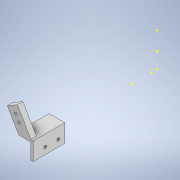
# Autodesk Inventor part: Bracket
Saved by Autodesk Inventor 2020.2 (Build 242310000, 310)
## iProperties
Created: 2020-10-07
Part Number: Bracket
Material: Generic
Document SubType Name: Modeling
Designer: Owner
Density: 1 g/cm^3
Appearance: Default
Author: Owner
Autodesk Inventor part; units mm, degrees
ref_plane "YZ Plane" through (0, 0, 0) normal (1, 0, 0) x (0, 1, 0)
ref_plane "XZ Plane" through (0, 0, 0) normal (0, 1, 0) x (-1, 0, 0)
ref_plane "XY Plane" through (0, 0, 0) normal (0, 0, 1) x (1, 0, 0)
sketch "Sketch1" plane through (0, 0, 0) normal (0, 0, 1) x (1, 0, 0)
  line L0 (0, 0) -> (19.05, 0)
  line L1 (19.05, 0) -> (19.05, 19.05)
  line L2 (19.05, 19.05) -> (0, 19.05)
  line L3 (0, 19.05) -> (0, 0)
  line L4 (19.05, 0) -> (22.225, 0)
  line L5 (22.225, 0) -> (22.225, 19.05)
  line L6 (22.225, 19.05) -> (19.05, 19.05)
  line L7 (19.05, 19.05) -> (19.05, 0)
  line L8 (0, 19.05) -> (22.225, 19.05)
  line L9 (22.225, 19.05) -> (22.225, 22.225)
  line L10 (22.225, 22.225) -> (0, 22.225)
  line L11 (0, 22.225) -> (0, 19.05)
  line L12 (0, 19.05) -> (-127, 19.05)
  line L13 (-127, 19.05) -> (-127, 22.225)
  line L14 (-127, 22.225) -> (0, 22.225)
  line L15 (0, 22.225) -> (0, 19.05)
  dimension "d0" = 19.05
  dimension "d1" = 19.05
  dimension "d2" = 3.175
  dimension "d3" = 3.175
  dimension "d4" = 127
  constraints: 32 end point, 8 parallel, 4 horizontal, 4 perpendicular, 2 point on line
  measures "d0" distance of L2.end L1.end
  measures "d1" distance of L1.end L0.end
  measures "d2" distance of L6.end L5.end
  measures "d3" distance of L9.end L8.end
  measures "d4" distance of L13.end L14.end
extrude "Extrusion1" add sketch "Sketch1" along normal blind 196.85 contours L1 L6 L5 L4 | L11 L10 L9 L6 L2 | L12 L13 L14 L11
sketch "Sketch2" plane through (-127, 22.225, 0) normal (0, 1, 0) x (1, 0, 0)
  line L0 (0, 0) -> (127, 0)
  line L1 (127, 0) -> (127, -34.925)
  line L2 (127, -34.925) -> (0, -34.925)
  line L3 (0, -34.925) -> (0, 0)
  dimension "d7" = 34.925
  constraints: 8 end point, 2 parallel, 1 horizontal, 1 perpendicular
  measures "d7" distance of L0.end L1.end
extrude "Extrusion2" cut sketch "Sketch2" against normal blind 25.4
sketch "Sketch3" plane through (-127, 22.225, 196.85) normal (0, 1, 0) x (1, 0, 0)
  line L0 (127, 161.925) -> (0, 161.925) projected
  line L1 (0, 161.925) -> (127, 161.925)
  line L2 (127, 161.925) -> (127, 158.75)
  line L3 (127, 158.75) -> (0, 158.75)
  line L4 (0, 158.75) -> (0, 161.925)
  point P0 (127, 196.85)
  dimension "d10" = 3.175
  constraints: 8 end point, 2 parallel, 1 horizontal, 1 perpendicular
  measures "d10" distance of L1.end L2.end
extrude "Extrusion3" add sketch "Sketch3" along normal blind 25.4
sketch "Sketch4" plane through (-127, 22.225, 196.85) normal (0, 1, 0) x (1, 0, 0)
  line L0 (149.225, 196.85) -> (127, 196.85) projected
  line L1 (149.225, 196.85) -> (149.225, 0) projected
  line L2 (127, 196.85) -> (149.225, 196.85)
  line L3 (149.225, 196.85) -> (149.225, 0)
  line L4 (149.225, 0) -> (127, 0)
  line L5 (127, 0) -> (127, 196.85)
  line L6 (149.225, 0) -> (0, 0) projected
  line L7 (138.1125, 0) -> (138.1125, 196.85)
  line L8 (127, 34.925) -> (149.225, 34.925)
  line L9 (127, 34.925) -> (149.225, 0)
  line L10 (127, 0) -> (149.225, 34.925)
  line L11 (127, 10.3909) -> (149.225, 24.5341)
  line L12 (127, 24.5341) -> (149.225, 10.3909)
  line L13 (127, 196.85) -> (127, 161.925) projected
  line L14 (127, 161.925) -> (149.225, 161.925)
  line L15 (127, 161.925) -> (149.225, 196.85)
  line L16 (149.225, 161.925) -> (127, 196.85)
  line L17 (127, 196.85) -> (127, 172.3159)
  line L18 (149.225, 186.4591) -> (127, 172.3159)
  line L19 (149.225, 172.3159) -> (127, 186.4591)
  line L20 (127, 186.4591) -> (149.225, 186.4591)
  line L21 (127, 10.3909) -> (149.225, 10.3909)
  line L22 (127, 172.3159) -> (149.225, 172.3159)
  line L23 (127, 24.5341) -> (149.225, 24.5341)
  circle A0 centre (138.1125, 10.3909) radius 1.905
  circle A1 centre (138.1125, 24.5341) radius 1.905
  circle A2 centre (138.1125, 172.3159) radius 1.905
  circle A3 centre (138.1125, 186.4591) radius 1.905
  dimension "d13" = 3.81
  dimension "d14" = 3.81
  dimension "d15" = 3.81
  dimension "d16" = 3.81
  constraints: 40 end point, 12 point on line, 11 perpendicular, 5 midpoint, 4 centre point, 3 parallel, 2 horizontal
  measures "d13" diameter of A0
  measures "d14" diameter of A1
  measures "d15" diameter of A2
  measures "d16" diameter of A3
extrude "Extrusion4" cut sketch "Sketch4" against normal blind 25.4 contours A3 L20 L7 | L7 L20 A3 | A3 L7 L20 | L7 A3 L20 | A2 L22 L7 | L7 L22 A2 | A2 L7 L22 | L7 A2 L22 | A1 L23 L7 | L7 L23 A1 | A1 L7 L23 | A0 L21 L7 | L7 L21 A0 | A1 L23 L7 | A0 L7 L21 | L7 A0 L21
sketch "Sketch5" plane through (22.225, 0, 0) normal (1, 0, 0) x (0, 0, -1)
  line L0 (0, 22.225) -> (-196.85, 22.225) projected
  line L1 (0, 0) -> (-196.85, 0) projected
  line L2 (-34.925, 22.225) -> (0, 22.225)
  line L3 (0, 22.225) -> (0, 0)
  line L4 (0, 0) -> (-34.925, 0)
  line L5 (-34.925, 0) -> (-34.925, 22.225)
  line L6 (-196.85, 22.225) -> (-161.925, 22.225)
  line L7 (-161.925, 22.225) -> (-161.925, 0)
  line L8 (-161.925, 0) -> (-196.85, 0)
  line L9 (-196.85, 0) -> (-196.85, 22.225)
  line L10 (-196.85, 19.05) -> (-196.85, 0) projected
  line L11 (-196.85, 11.1125) -> (0, 11.1125)
  line L12 (0, 19.05) -> (0, 0) projected
  line L13 (0, 22.225) -> (-34.925, 0)
  line L14 (-34.925, 22.225) -> (0, 0)
  line L15 (-196.85, 22.225) -> (-161.925, 0)
  line L16 (-161.925, 22.225) -> (-196.85, 0)
  line L17 (-186.4591, 22.225) -> (-172.3159, 0)
  line L18 (-174.2209, 22.225) -> (-170.4109, 22.225) projected
  line L19 (-172.3159, 22.225) -> (-186.4591, 0)
  line L20 (-24.4964, 22.225) -> (-10.3532, 0)
  line L21 (-10.3532, 22.225) -> (-24.4964, 0)
  line L22 (-24.4964, 22.225) -> (-24.4964, 0)
  line L23 (-10.3532, 22.225) -> (-10.3532, 0)
  line L24 (-186.4591, 22.225) -> (-186.4591, 0)
  line L25 (-172.3159, 22.225) -> (-172.3159, 0)
  circle A0 centre (-186.4591, 11.1125) radius 1.905
  circle A1 centre (-172.3159, 11.1125) radius 1.905
  circle A2 centre (-24.4964, 11.1125) radius 1.905
  dimension "d19" = 34.925
  dimension "d20" = 3.81
  dimension "d21" = 3.81
  dimension "d22" = 3.81
  constraints: 42 end point, 12 point on line, 11 parallel, 6 perpendicular, 4 midpoint, 3 centre point, 2 horizontal
  measures "d19" distance of L7.end L8.end
  measures "d20" diameter of A0
  measures "d21" diameter of A1
  measures "d22" diameter of A2
extrude "Extrusion5" cut sketch "Sketch5" against normal blind 25.4 contours A2 L11 L22 | L22 L11 A2 | L11 L22 A2 | A2 L22 L11 | A1 L25 L11 | L11 L25 A1 | L25 L11 A1 | L25 A1 L11 | A0 L24 L11 | L11 L24 A0 | L24 A0 L11 | L11 A0 L24
sketch "Sketch6" plane through (22.225, 0, 0) normal (1, 0, 0) x (0, 0, -1)
  line L0 (0, 22.225) -> (-196.85, 22.225) projected
  line L1 (0, 19.05) -> (0, 0) projected
  line L2 (-34.4902, 22.225) -> (0, 22.225)
  line L3 (0, 22.225) -> (0, 0)
  line L4 (0, 0) -> (-34.4902, 0)
  line L5 (-34.4902, 0) -> (-34.4902, 22.225)
  line L6 (-34.4902, 11.1125) -> (0, 11.1125)
  line L7 (0, 0) -> (0, 22.225) projected
  line L8 (0, 22.225) -> (-34.4902, 0)
  line L9 (-24.4058, 22.225) -> (-10.0843, 0)
  line L10 (0, 0) -> (-196.85, 0) projected
  line L11 (-10.0843, 0) -> (-10.0843, 22.225)
  circle A0 centre (-10.0843, 11.1125) radius 1.905
  dimension "d25" = 3.81
  constraints: 16 end point, 4 point on line, 3 midpoint, 3 perpendicular, 2 parallel, 1 centre point, 1 horizontal
  measures "d25" diameter of A0
extrude "Extrusion6" cut sketch "Sketch6" against normal blind 25.4 contours A0 L6 L11 | L11 L6 A0 | A0 L11 L6 | L6 L11 A0
sketch "Sketch7" plane through (0, 19.05, 34.925) normal (0, 0, -1) x (-1, 0, 0)
  point P0 (0, -19.05)
sketch "Sketch8" plane through (0, 19.05, 34.925) normal (0, 0, -1) x (-1, 0, 0)
  line L0 (0, 28.575) -> (127, 28.575) projected
  line L1 (0, 3.3903) -> (127, 3.3903)
  line L2 (127, 3.3903) -> (127, 28.575)
  line L3 (127, 28.575) -> (0, 28.575)
  line L4 (0, 28.575) -> (0, 3.3903)
  point P0 (0, -19.05)
  constraints: 8 end point, 2 parallel, 1 horizontal, 1 perpendicular
extrude "Extrusion7" cut sketch "Sketch8" against normal blind 25.4
sketch "Sketch9" plane through (-127, 22.225, 196.85) normal (0, 1, 0) x (1, 0, 0)
  point P0 (127, 196.85)
sketch "Sketch10" plane through (0, 19.05, 34.925) normal (0, 0, -1) x (-1, 0, 0)
  line L0 (0, 3.175) -> (0, 0) projected
  line L1 (0, 0) -> (127, 0)
  line L2 (127, 0) -> (127, 3.175)
  line L3 (127, 3.175) -> (0, 3.175)
  line L4 (0, 3.175) -> (0, 0)
  point P0 (0, -19.05)
  constraints: 8 end point, 2 parallel, 1 horizontal, 1 perpendicular
extrude "Extrusion8" cut sketch "Sketch10" against normal blind 184.15
sketch "Sketch11" plane through (0, 22.4403, 34.925) normal (0, 0, -1) x (-1, 0, 0)
  point P0 (0, -22.4403)
sketch "Sketch12" plane through (0, 22.4403, 34.925) normal (0, 0, -1) x (-1, 0, 0)
  line L0 (0, -3.3903) -> (0, -0.2153) projected
  line L1 (0, -3.3903) -> (693.4588, -3.3903)
  line L2 (693.4588, -3.3903) -> (693.4588, 311.9372)
  line L3 (693.4588, 311.9372) -> (0, 311.9372)
  line L4 (0, 311.9372) -> (0, -3.3903)
  point P0 (0, -22.4403)
  constraints: 8 end point, 2 parallel, 1 horizontal, 1 perpendicular
extrude "Extrusion9" cut sketch "Sketch12" against normal blind 25.4
sketch "Sketch13" plane through (0, 22.225, 0) normal (-1, 0, 0) x (0, 0, 1)
  line L0 (0, 0) -> (196.85, 0) projected
  line L1 (196.85, -3.175) -> (0, -3.175)
  line L2 (0, -3.175) -> (0, 0)
  line L3 (0, 0) -> (196.85, 0)
  line L4 (196.85, 0) -> (196.85, -3.175)
  point P0 (0, -22.225)
  constraints: 8 end point, 2 parallel, 1 horizontal, 1 perpendicular
extrude "Extrusion10" add sketch "Sketch13" along normal blind 127
sketch "Sketch14" plane through (22.225, 22.225, 196.85) normal (0, 1, 0) x (1, 0, 0)
  line L0 (-149.225, 196.85) -> (-149.225, 0) projected
  line L1 (-149.225, 0) -> (0.7773, 0)
  line L2 (0.7773, 0) -> (0.7773, -19.05)
  line L3 (0.7773, -19.05) -> (-149.225, -19.05)
  line L4 (-149.225, -19.05) -> (-149.225, 0)
  line L5 (-149.225, -19.05) -> (0.7773, -19.05)
  line L6 (0.7773, -19.05) -> (0.7773, -21.336)
  line L7 (0.7773, -21.336) -> (-149.225, -21.336)
  line L8 (-149.225, -21.336) -> (-149.225, -19.05)
  line L9 (0, 196.85) -> (0, 0) projected
  line L10 (-149.225, -19.05) -> (0, -19.05)
  line L11 (0, -19.05) -> (0, 4.95)
  line L12 (0, 4.95) -> (-149.225, 4.95)
  line L13 (-149.225, 4.95) -> (-149.225, -19.05)
  line L14 (-149.225, 4.95) -> (0, 4.95)
  line L15 (0, 4.95) -> (0, 55.75)
  line L16 (0, 55.75) -> (-149.225, 55.75)
  line L17 (-149.225, 55.75) -> (-149.225, 4.95)
  line L18 (-149.225, 55.75) -> (0, 55.75)
  line L19 (0, 55.75) -> (0, 176.4)
  line L20 (0, 176.4) -> (-149.225, 176.4)
  line L21 (-149.225, 176.4) -> (-149.225, 55.75)
  line L22 (-149.225, 176.4) -> (-22.225, 176.4)
  line L23 (-22.225, 176.4) -> (-22.225, 179.575)
  line L24 (-22.225, 179.575) -> (-149.225, 179.575)
  line L25 (-149.225, 179.575) -> (-149.225, 176.4)
  point P0 (-22.225, 196.85)
  dimension "d36" = 19.05
  dimension "d37" = 2.286
  dimension "d38" = 24
  dimension "d39" = 50.8
  dimension "d40" = 120.65
  dimension "d41" = 3.175
  constraints: 48 end point, 12 parallel, 6 horizontal, 6 perpendicular, 4 point on line
  measures "d36" distance of L1.end L2.end
  measures "d37" distance of L5.end L6.end
  measures "d38" distance of L11.end L10.end
  measures "d39" distance of L15.end L14.end
  measures "d40" distance of L19.end L18.end
  measures "d41" distance of L23.end L22.end
extrude "Extrusion11" add sketch "Sketch14" along normal blind 25.4 contours L24 L23 L20 L0
sketch "Sketch16" plane through (22.225, 22.225, 196.85) normal (0, 1, 0) x (1, 0, 0)
  line L0 (-3.175, 196.85) -> (-3.175, 0) projected
  line L1 (-3.175, 0) -> (-41.275, 0)
  line L2 (-41.275, 0) -> (-41.275, 7.6439)
  line L3 (-41.275, 7.6439) -> (-3.175, 7.6439)
  line L4 (-3.175, 7.6439) -> (-3.175, 0)
  point P0 (-22.225, 196.85)
  point P1 (-3.175, 7.6439)
  dimension "d48" = 38.1
  constraints: 8 end point, 2 parallel, 1 horizontal, 1 perpendicular
  measures "d48" distance of L2.end L3.end
extrude "Extrusion12" add sketch "Sketch16" along normal blind 32.9946
sketch "Sketch17" plane through (0, 0, 196.85) normal (0, 0, 1) x (1, 0, 0)
  line L0 (19.05, 55.2196) -> (-19.05, 55.2196) projected
  line L1 (0, 22.225) -> (0, 47.625) projected
  line L2 (0, 55.2196) -> (0, 22.225)
  line L3 (19.05, 22.225) -> (19.05, 55.2196) projected
  line L4 (19.05, 55.2196) -> (0, 55.2196)
  line L5 (0, 55.2196) -> (0, 22.225)
  line L6 (0, 22.225) -> (19.05, 22.225)
  line L7 (19.05, 22.225) -> (19.05, 55.2196)
  line L8 (-19.05, 55.2196) -> (0, 55.2196)
  line L9 (0, 55.2196) -> (0, 22.225)
  line L10 (0, 22.225) -> (-19.05, 22.225)
  line L11 (-19.05, 22.225) -> (-19.05, 55.2196)
  line L12 (-19.05, 55.2196) -> (0, 22.225)
  line L13 (0, 55.2196) -> (19.05, 22.225)
  line L14 (0, 55.2196) -> (-14.2873, 46.9706)
  point P0 (0, 0)
  constraints: 24 end point, 5 parallel, 3 perpendicular, 2 horizontal, 1 midpoint, 1 point on line, 1 vertical
extrude "Extrusion13" cut sketch "Sketch17" against normal blind 25.4 contours L3 L13 L0 | L14 L12 L0 | L12 L10 L11
sketch "Sketch18" plane through (22.225, 22.225, 196.85) normal (0, 1, 0) x (1, 0, 0)
  line L0 (-3.175, 196.85) -> (-3.175, 0) projected
  line L1 (-3.175, 196.85) -> (-41.275, 196.85)
  line L2 (-41.275, 196.85) -> (-41.275, 189.23)
  line L3 (-41.275, 189.23) -> (-3.175, 189.23)
  line L4 (-3.175, 189.23) -> (-3.175, 196.85)
  point P0 (-22.225, 196.85)
  point P1 (-3.175, 189.23)
  dimension "d53" = 38.1
  dimension "d54" = 7.62
  constraints: 8 end point, 2 parallel, 1 horizontal, 1 perpendicular
  measures "d53" distance of L3.end L2.end
  measures "d54" distance of L2.end L1.end
extrude "Extrusion14" add sketch "Sketch18" along normal blind 32.9946
sketch "Sketch19" plane through (0, 0, 0) normal (0, 0, -1) x (-1, 0, 0)
  line L0 (0, 22.225) -> (0, 47.625) projected
  line L1 (19.05, 55.2196) -> (-19.05, 55.2196) projected
  line L2 (0, 22.225) -> (-19.05, 22.225)
  line L3 (-19.05, 22.225) -> (-19.05, 55.2196)
  line L4 (-19.05, 55.2196) -> (0, 55.2196)
  line L5 (0, 55.2196) -> (0, 22.225)
  line L6 (19.05, 55.2196) -> (0, 55.2196)
  line L7 (0, 55.2196) -> (0, 22.225)
  line L8 (0, 22.225) -> (19.05, 22.225)
  line L9 (19.05, 22.225) -> (19.05, 55.2196)
  line L10 (19.05, 22.225) -> (19.05, 55.2196) projected
  line L11 (19.05, 55.2196) -> (0, 22.225)
  line L12 (0, 55.2196) -> (-19.05, 22.225)
  line L13 (14.2873, 46.9706) -> (0, 55.2196) projected
  line L14 (14.2873, 46.9706) -> (0, 55.2196)
  point P0 (0, 0)
  constraints: 22 end point, 6 equal length, 2 horizontal, 2 perpendicular
extrude "Extrusion15" cut sketch "Sketch19" against normal blind 10.16 contours L11 L9 L8 | L3 L1 L12 | L13 L1 L11
sketch "Sketch21" plane through (0, 0, 196.85) normal (0, 0, 1) x (1, 0, 0)
  line L0 (0, 22.225) -> (-127, 22.225) projected
  line L1 (0, 55.392) -> (0, 22.225)
  line L2 (-14.2873, 46.9706) -> (0, 22.225) projected
  line L3 (0, 22.225) -> (14.2873, 30.474)
  line L4 (19.05, 22.225) -> (0, 55.2196) projected
  line L5 (-14.3754, 47.2229) -> (14.2873, 30.474)
  line L6 (0, 55.2196) -> (-14.2873, 46.9706) projected
  line L7 (-7.1436, 51.0951) -> (7.1436, 26.3495)
  line L8 (-4.9375, 30.5073) -> (4.8012, 47.1733)
  line L9 (4.8012, 47.1733) -> (-9.6604, 38.8237)
  line L10 (-9.6604, 38.8237) -> (9.4665, 38.8237)
  line L11 (9.4665, 38.8237) -> (-4.9375, 30.5073)
  circle A0 centre (-2.4296, 42.9985) radius 1.905
  circle A1 centre (2.2645, 34.6655) radius 1.905
  point P0 (0, 0)
  dimension "d63" = 3.81
  dimension "d64" = 3.81
  constraints: 16 end point, 4 midpoint, 3 perpendicular, 2 centre point, 1 horizontal, 1 point on line, 1 vertical
  measures "d63" diameter of A0
  measures "d64" diameter of A1
extrude "Extrusion16" cut sketch "Sketch21" against normal blind 203.2 contours A0 L7 L9 | L9 L7 A0 | L7 L9 A0 | L7 A0 L9 | A1 L11 L7 | L7 L11 A1 | A1 L7 L11 | L11 L7 A1
sketch "Sketch22" plane through (-127, 22.225, 20.45) normal (0, 0, 1) x (1, 0, 0)
  line L0 (126.5097, 23.8424) -> (122.0809, 23.8424)
  line L1 (122.0809, 23.8424) -> (122.0809, 18.1325)
  line L2 (122.0809, 18.1325) -> (126.5097, 18.1325)
  line L3 (126.5097, 18.1325) -> (126.5097, 23.8424)
  point P0 (127, -22.225)
  constraints: 8 end point, 2 parallel, 1 horizontal, 1 perpendicular
extrude "Extrusion17" add sketch "Sketch22" against normal blind 3.81
sketch "Sketch23" plane through (22.225, 47.625, 196.85) normal (0, 1, 0) x (1, 0, 0)
  point P0 (-22.225, 196.85)
sketch "Sketch24" plane through (22.225, 47.625, 196.85) normal (0, 1, 0) x (1, 0, 0)
  line L0 (-37.6865, 183.5382) -> (-20.0753, 183.5382)
  line L1 (-20.0753, 183.5382) -> (-20.0753, 172.2108)
  line L2 (-20.0753, 172.2108) -> (-37.6865, 172.2108)
  line L3 (-37.6865, 172.2108) -> (-37.6865, 183.5382)
  point P0 (-22.225, 196.85)
  constraints: 8 end point, 2 parallel, 1 horizontal, 1 perpendicular
extrude "Extrusion18" cut sketch "Sketch24" against normal blind 25.4
sketch "Sketch25" plane through (22.225, 47.625, 196.85) normal (0, 1, 0) x (1, 0, 0)
  line L0 (-149.225, 196.85) -> (-149.225, 0) projected
  line L1 (-149.225, 171.0005) -> (-36.4868, 171.0005)
  line L2 (-36.4868, 171.0005) -> (-36.4868, 186.4508)
  line L3 (-36.4868, 186.4508) -> (-149.225, 186.4508)
  line L4 (-149.225, 186.4508) -> (-149.225, 171.0005)
  point P0 (-22.225, 196.85)
  constraints: 8 end point, 2 parallel, 1 horizontal, 1 perpendicular, 1 point on line
extrude "Extrusion19" cut sketch "Sketch25" against normal blind 25.4
sketch "Sketch26" plane through (22.225, 22.225, 196.85) normal (0, 1, 0) x (1, 0, 0)
  line L0 (-36.5123, 189.23) -> (-22.225, 189.23) projected
  line L1 (-149.225, 196.85) -> (-36.5123, 196.85)
  line L2 (-36.5123, 196.85) -> (-36.5123, 189.23)
  line L3 (-36.5123, 189.23) -> (-149.225, 189.23)
  line L4 (-149.225, 189.23) -> (-149.225, 196.85)
  line L5 (-22.225, 196.85) -> (-36.5123, 196.85) projected
  line L6 (-36.5123, 189.23) -> (-22.225, 196.85)
  line L7 (-22.225, 196.85) -> (-36.5123, 196.85)
  line L8 (-36.5123, 196.85) -> (-22.225, 189.23)
  line L9 (-22.225, 196.85) -> (-22.225, 189.23) projected
  line L10 (-36.5123, 189.23) -> (-22.225, 189.23)
  line L11 (-22.225, 189.23) -> (-22.225, 193.04)
  line L12 (-22.225, 193.04) -> (-36.5123, 193.04)
  line L13 (-36.5123, 193.04) -> (-36.5123, 189.23)
  line L14 (-36.5123, 196.85) -> (-22.225, 196.85)
  line L15 (-22.225, 196.85) -> (-22.225, 193.04)
  line L16 (-22.225, 193.04) -> (-36.5123, 193.04)
  line L17 (-36.5123, 193.04) -> (-36.5123, 196.85)
  line L18 (-36.5123, 191.135) -> (-22.225, 191.135)
  line L19 (-36.5123, 194.945) -> (-22.225, 194.945)
  line L20 (-36.5123, 191.135) -> (-22.225, 191.135)
  line L21 (-22.225, 191.135) -> (-22.225, 194.945)
  line L22 (-22.225, 194.945) -> (-36.5123, 194.945)
  line L23 (-36.5123, 194.945) -> (-36.5123, 191.135)
  constraints: 42 end point, 9 equal length, 5 midpoint, 4 horizontal, 4 perpendicular
extrude "Extrusion20" add sketch "Sketch26" along normal blind 25.4 fills toward (-92.8686, 189.28) open curves L3 L4 L1
sketch "Sketch27" plane through (-127, 22.225, 7.62) normal (0, 0, 1) x (1, 0, 0)
  point P0 (127, -22.225)
sketch "Sketch28" plane through (0, 0, 0) normal (0, 0, -1) x (-1, 0, 0)
  point P0 (0, 0)
sketch "Sketch29" plane through (-127, 22.225, 7.62) normal (0, 0, 1) x (1, 0, 0)
  line L0 (0, 0) -> (148.1919, 0)
  line L1 (148.1919, 0) -> (148.1919, 42.5279)
  line L2 (148.1919, 42.5279) -> (0, 42.5279)
  line L3 (0, 42.5279) -> (0, 0)
  point P0 (127, -22.225)
  constraints: 8 end point, 2 parallel, 1 horizontal, 1 perpendicular
extrude "Extrusion21" cut sketch "Sketch29" against normal blind 2.54
sketch "Sketch30" plane through (0, 0, 0) normal (0, 0, -1) x (-1, 0, 0)
  line L0 (-41.7951, 65.3416) -> (150.992, 65.3416)
  line L1 (150.992, 65.3416) -> (150.992, -18.2485)
  line L2 (150.992, -18.2485) -> (-41.7951, -18.2485)
  line L3 (-41.7951, -18.2485) -> (-41.7951, 65.3416)
  point P0 (0, 0)
  constraints: 8 end point, 2 parallel, 1 horizontal, 1 perpendicular
extrude "Extrusion22" cut sketch "Sketch30" against normal blind 152.4
sketch "Sketch31" plane through (0, 0, 152.4) normal (0, 0, -1) x (-1, 0, 0)
  line L0 (0, 55.2196) -> (14.2873, 46.9706) projected
  line L1 (14.2873, 46.9706) -> (-5.2989, 13.0463)
  line L2 (14.2873, 46.9706) -> (53.4597, 46.9706) construction
  line L3 (-5.2989, 13.0463) -> (139.7287, 9.4303)
  line L4 (139.7287, 9.4303) -> (128.1209, 43.3923)
  line L5 (128.1209, 43.3923) -> (14.2873, 46.9706)
  point P0 (0, 0)
  dimension "d80" = 120
  constraints: 10 end point, 1 equal length, 1 horizontal
  measures "d80" angle of L1 L2
extrude "Extrusion23" cut sketch "Sketch31" against normal blind 50.8
sketch "Sketch32" plane through (22.225, 0, 196.85) normal (1, 0, 0) x (0, 0, -1)
  line L0 (27.9081, 15.5282) -> (19.6428, 15.5282)
  line L1 (19.6428, 15.5282) -> (19.6428, 5.1445)
  line L2 (19.6428, 5.1445) -> (27.9081, 5.1445)
  line L3 (27.9081, 5.1445) -> (27.9081, 15.5282)
  line L4 (13.6349, 16.0143) -> (6.0295, 16.0143)
  line L5 (6.0295, 16.0143) -> (6.0295, 5.8391)
  line L6 (6.0295, 5.8391) -> (13.6349, 5.8391)
  line L7 (13.6349, 5.8391) -> (13.6349, 16.0143)
  point P0 (196.85, 0)
  constraints: 16 end point, 4 parallel, 2 horizontal, 2 perpendicular
extrude "Extrusion24" add sketch "Sketch32" against normal blind 3.175
sketch "Sketch33" plane through (22.225, 0, 196.85) normal (1, 0, 0) x (0, 0, -1)
  line L0 (0, 0) -> (0, 22.225) projected
  line L1 (44.45, 19.05) -> (0, 19.05) projected
  line L2 (0, 22.225) -> (44.45, 22.225)
  line L3 (44.45, 22.225) -> (44.45, 19.05)
  line L4 (44.45, 19.05) -> (0, 19.05)
  line L5 (0, 19.05) -> (0, 22.225)
  line L6 (44.45, 19.05) -> (44.45, 0) projected
  line L7 (0, 19.05) -> (44.45, 19.05)
  line L8 (44.45, 19.05) -> (44.45, 15.875)
  line L9 (44.45, 15.875) -> (0, 15.875)
  line L10 (0, 15.875) -> (0, 19.05)
  line L11 (0, 15.875) -> (44.45, 15.875)
  line L12 (44.45, 15.875) -> (44.45, -3.175)
  line L13 (44.45, -3.175) -> (0, -3.175)
  line L14 (0, -3.175) -> (0, 15.875)
  line L15 (7.6439, 22.225) -> (7.6439, 46.9706) projected
  line L16 (7.6439, 25.7053) -> (7.6439, -11.462)
  line L17 (7.6439, 15.875) -> (44.45, -3.175)
  line L18 (7.6439, -3.175) -> (44.45, 15.875)
  line L19 (26.047, 15.875) -> (26.047, -5.3743)
  line L20 (7.6439, -3.175) -> (26.047, 15.875)
  line L21 (7.6439, 15.875) -> (26.047, -3.175)
  line L22 (26.047, 15.875) -> (44.45, -3.175)
  line L23 (44.45, 15.875) -> (26.047, -3.175)
  circle A0 centre (16.8454, 6.35) radius 1.905
  circle A1 centre (35.2485, 6.35) radius 1.905
  point P0 (196.85, 0)
  dimension "d85" = 3.175
  dimension "d86" = 3.175
  dimension "d87" = 19.05
  dimension "d88" = 3.81
  dimension "d89" = 3.81
  constraints: 40 end point, 9 point on line, 6 parallel, 3 horizontal, 3 perpendicular, 2 centre point, 2 midpoint, 2 vertical
  measures "d85" distance of L2.end L1.start
  measures "d86" distance of L7.end L8.end
  measures "d87" distance of L11.end L12.end
  measures "d88" diameter of A0
  measures "d89" diameter of A1
extrude "Extrusion25" cut sketch "Sketch33" against normal blind 3.81 contours A0 L20 L21 | L21 L20 A0 | L20 L21 A0 | A0 L21 L20 | A1 L22 L23 | L23 L22 A1 | L22 L23 A1 | A1 L23 L22
sketch "Sketch34" plane through (22.225, 0, 196.85) normal (1, 0, 0) x (0, 0, -1)
  line L0 (0, 0) -> (0, 22.225) projected
  line L1 (44.45, 19.05) -> (0, 19.05) projected
  line L2 (0, 22.225) -> (44.45, 22.225)
  line L3 (44.45, 22.225) -> (44.45, 19.05)
  line L4 (44.45, 19.05) -> (0, 19.05)
  line L5 (0, 19.05) -> (0, 22.225)
  line L6 (44.45, 19.05) -> (44.45, 0) projected
  line L7 (0, 19.05) -> (44.45, 19.05)
  line L8 (44.45, 19.05) -> (44.45, 15.875)
  line L9 (44.45, 15.875) -> (0, 15.875)
  line L10 (0, 15.875) -> (0, 19.05)
  line L11 (0, 15.875) -> (44.45, 15.875)
  line L12 (44.45, 15.875) -> (44.45, -3.175)
  line L13 (44.45, -3.175) -> (0, -3.175)
  line L14 (0, -3.175) -> (0, 15.875)
  line L15 (0, 19.05) -> (0, 0) projected
  line L16 (0, 0) -> (44.45, 0)
  line L17 (44.45, 0) -> (44.45, -3.175)
  line L18 (44.45, -3.175) -> (0, -3.175)
  line L19 (0, -3.175) -> (0, 0)
  point P0 (196.85, 0)
  dimension "d92" = 3.175
  dimension "d93" = 3.175
  dimension "d94" = 19.05
  constraints: 32 end point, 8 parallel, 4 horizontal, 4 perpendicular, 2 point on line
  measures "d92" distance of L2.end L1.start
  measures "d93" distance of L7.end L8.end
  measures "d94" distance of L11.end L12.end
extrude "Extrusion26" add sketch "Sketch34" against normal blind 3.175 contours L16 L12 L13 L14
sketch "Sketch35" plane through (0, 22.225, 189.2061) normal (0, 1, 0) x (1, 0, 0)
  line L0 (1.8327, -7.6439) -> (1.8327, 36.8061) projected
  line L1 (20.288, 28.1094) -> (1.8327, 28.1094)
  line L2 (1.8327, 28.1094) -> (1.8327, 0.5756)
  line L3 (1.8327, 0.5756) -> (20.288, 0.5756)
  line L4 (20.288, 0.5756) -> (20.288, 28.1094)
  point P0 (0, 189.2061)
  point P1 (1.8327, 28.1094)
  constraints: 8 end point, 2 parallel, 1 horizontal, 1 perpendicular, 1 point on line
extrude "Extrusion27" add sketch "Sketch35" against normal blind 3.175
equation "\"d90\" = d89"
body "Solid1"
